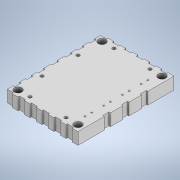
# Autodesk Inventor part: TOP_PANEL
Saved by Autodesk Inventor 2020.4 (Build 244396010, 396A)
## iProperties
Created: 2021-10-02
Part Number: TOP_PANEL
Material: Generic
Document SubType Name: Modeling
Designer: YUSTE
Density: 1 g/cm^3
Appearance: Default
Author: YUSTE
Autodesk Inventor part; units mm, degrees
ref_plane "YZ Plane" through (0, 0, 0) normal (1, 0, 0) x (0, 1, 0)
ref_plane "XZ Plane" through (0, 0, 0) normal (0, 1, 0) x (-1, 0, 0)
ref_plane "XY Plane" through (0, 0, 0) normal (0, 0, 1) x (1, 0, 0)
sketch "Sketch1" plane through (0, 0, 0) normal (0, 1, 0) x (-1, 0, 0)
  line L0 (0, 0) -> (152.4, 0)
  line L1 (152.4, 0) -> (152.4, 203.2)
  line L2 (152.4, 203.2) -> (0, 203.2)
  line L3 (0, 203.2) -> (0, 0)
  circle A0 centre (12.7, 190.5) radius 7.9375
  circle A1 centre (139.7, 190.5) radius 7.9375
  circle A2 centre (139.7, 12.7) radius 7.9375
  circle A3 centre (12.7, 12.7) radius 7.9375
  circle A4 centre (114.3, 190.5) radius 3.302
  circle A5 centre (38.1, 190.5) radius 3.302
  circle A6 centre (114.3, 12.7) radius 3.302
  circle A7 centre (38.1, 12.7) radius 3.302
  circle A8 centre (139.7, 139.7) radius 3.302
  circle A9 centre (139.7, 63.5) radius 3.302
  circle A10 centre (20.32, 168.148) radius 1.524
  circle A11 centre (20.32, 153.924) radius 1.524
  circle A12 centre (20.32, 128.524) radius 1.524
  circle A13 centre (20.32, 114.3) radius 1.524
  circle A14 centre (20.32, 88.9) radius 1.524
  circle A15 centre (20.32, 74.676) radius 1.524
  circle A16 centre (20.32, 49.276) radius 1.524
  circle A17 centre (20.32, 35.052) radius 1.524
  line L4 (152.4, 203.2) -> (139.7, 203.2)
  line L5 (139.7, 203.2) -> (139.7, 200.025)
  line L6 (139.7, 200.025) -> (152.4, 200.025)
  line L7 (152.4, 200.025) -> (152.4, 203.2)
  line L8 (127, 203.2) -> (114.3, 203.2)
  line L9 (114.3, 203.2) -> (114.3, 200.025)
  line L10 (114.3, 200.025) -> (127, 200.025)
  line L11 (127, 200.025) -> (127, 203.2)
  line L12 (101.6, 203.2) -> (88.9, 203.2)
  line L13 (88.9, 203.2) -> (88.9, 200.025)
  line L14 (88.9, 200.025) -> (101.6, 200.025)
  line L15 (101.6, 200.025) -> (101.6, 203.2)
  line L16 (76.2, 203.2) -> (63.5, 203.2)
  line L17 (63.5, 203.2) -> (63.5, 200.025)
  line L18 (63.5, 200.025) -> (76.2, 200.025)
  line L19 (76.2, 200.025) -> (76.2, 203.2)
  line L20 (50.8, 203.2) -> (38.1, 203.2)
  line L21 (38.1, 203.2) -> (38.1, 200.025)
  line L22 (38.1, 200.025) -> (50.8, 200.025)
  line L23 (50.8, 200.025) -> (50.8, 203.2)
  line L24 (25.4, 203.2) -> (12.7, 203.2)
  line L25 (12.7, 203.2) -> (12.7, 200.025)
  line L26 (12.7, 200.025) -> (25.4, 200.025)
  line L27 (25.4, 200.025) -> (25.4, 203.2)
  line L28 (152.4, 0) -> (139.7, 0)
  line L29 (139.7, 0) -> (139.7, 3.175)
  line L30 (139.7, 3.175) -> (152.4, 3.175)
  line L31 (152.4, 3.175) -> (152.4, 0)
  line L32 (127, 0) -> (114.3, 0)
  line L33 (114.3, 0) -> (114.3, 3.175)
  line L34 (114.3, 3.175) -> (127, 3.175)
  line L35 (127, 3.175) -> (127, 0)
  line L36 (101.6, 0) -> (88.9, 0)
  line L37 (88.9, 0) -> (88.9, 3.175)
  line L38 (88.9, 3.175) -> (101.6, 3.175)
  line L39 (101.6, 3.175) -> (101.6, 0)
  line L40 (76.2, 0) -> (63.5, 0)
  line L41 (63.5, 0) -> (63.5, 3.175)
  line L42 (63.5, 3.175) -> (76.2, 3.175)
  line L43 (76.2, 3.175) -> (76.2, 0)
  line L44 (50.8, 0) -> (38.1, 0)
  line L45 (38.1, 0) -> (38.1, 3.175)
  line L46 (38.1, 3.175) -> (50.8, 3.175)
  line L47 (50.8, 3.175) -> (50.8, 0)
  line L48 (25.4, 0) -> (12.7, 0)
  line L49 (12.7, 0) -> (12.7, 3.175)
  line L50 (12.7, 3.175) -> (25.4, 3.175)
  line L51 (25.4, 3.175) -> (25.4, 0)
  line L52 (152.4, 187.325) -> (149.225, 187.325)
  line L53 (149.225, 187.325) -> (149.225, 174.625)
  line L54 (149.225, 174.625) -> (152.4, 174.625)
  line L55 (152.4, 174.625) -> (152.4, 187.325)
  line L56 (152.4, 161.925) -> (149.225, 161.925)
  line L57 (149.225, 161.925) -> (149.225, 149.225)
  line L58 (149.225, 149.225) -> (152.4, 149.225)
  line L59 (152.4, 149.225) -> (152.4, 161.925)
  line L60 (152.4, 136.525) -> (149.225, 136.525)
  line L61 (149.225, 136.525) -> (149.225, 123.825)
  line L62 (149.225, 123.825) -> (152.4, 123.825)
  line L63 (152.4, 123.825) -> (152.4, 136.525)
  line L64 (152.4, 107.95) -> (149.225, 107.95)
  line L65 (149.225, 107.95) -> (149.225, 95.25)
  line L66 (149.225, 95.25) -> (152.4, 95.25)
  line L67 (152.4, 95.25) -> (152.4, 107.95)
  line L68 (152.4, 79.375) -> (149.225, 79.375)
  line L69 (149.225, 79.375) -> (149.225, 66.675)
  line L70 (149.225, 66.675) -> (152.4, 66.675)
  line L71 (152.4, 66.675) -> (152.4, 79.375)
  line L72 (152.4, 53.975) -> (149.225, 53.975)
  line L73 (149.225, 53.975) -> (149.225, 41.275)
  line L74 (149.225, 41.275) -> (152.4, 41.275)
  line L75 (152.4, 41.275) -> (152.4, 53.975)
  line L76 (152.4, 28.575) -> (149.225, 28.575)
  line L77 (149.225, 28.575) -> (149.225, 15.875)
  line L78 (149.225, 15.875) -> (152.4, 15.875)
  line L79 (152.4, 15.875) -> (152.4, 28.575)
  line L80 (0, 147.574) -> (0, 134.874)
  line L81 (0, 134.874) -> (3.175, 134.874)
  line L82 (3.175, 134.874) -> (3.175, 147.574)
  line L83 (3.175, 147.574) -> (0, 147.574)
  line L84 (0, 107.95) -> (0, 95.25)
  line L85 (0, 95.25) -> (3.175, 95.25)
  line L86 (3.175, 95.25) -> (3.175, 107.95)
  line L87 (3.175, 107.95) -> (0, 107.95)
  line L88 (0, 55.626) -> (0, 68.326)
  line L89 (0, 68.326) -> (3.175, 68.326)
  line L90 (3.175, 68.326) -> (3.175, 55.626)
  line L91 (3.175, 55.626) -> (0, 55.626)
  dimension "d0" = 152.4
  dimension "d1" = 203.2
  dimension "d40" = 15.875
  dimension "d41" = 15.875
  dimension "d42" = 15.875
  dimension "d43" = 15.875
  dimension "d44" = 12.7
  dimension "d45" = 12.7
  dimension "d46" = 12.7
  dimension "d47" = 12.7
  dimension "d48" = 12.7
  dimension "d49" = 12.7
  dimension "d50" = 12.7
  dimension "d51" = 12.7
  dimension "d52" = 177.8
  dimension "d53" = 127
  dimension "d54" = 6.604
  dimension "d55" = 6.604
  dimension "d56" = 25.4
  dimension "d57" = 25.4
  dimension "d58" = 12.7
  dimension "d59" = 12.7
  dimension "d60" = 6.604
  dimension "d61" = 6.604
  dimension "d62" = 12.7
  dimension "d63" = 12.7
  dimension "d64" = 25.4
  dimension "d65" = 25.4
  dimension "d66" = 6.604
  dimension "d67" = 6.604
  dimension "d68" = 50.8
  dimension "d69" = 50.8
  dimension "d70" = 12.7
  dimension "d71" = 12.7
  dimension "d72" = 3.048
  dimension "d73" = 3.048
  dimension "d74" = 3.048
  dimension "d75" = 3.048
  dimension "d76" = 3.048
  dimension "d77" = 3.048
  dimension "d78" = 20.32
  dimension "d79" = 20.32
  dimension "d80" = 20.32
  dimension "d81" = 20.32
  dimension "d82" = 20.32
  dimension "d83" = 20.32
  dimension "d84" = 22.352
  dimension "d85" = 14.224
  dimension "d86" = 25.4
  dimension "d87" = 14.224
  dimension "d88" = 25.4
  dimension "d89" = 14.224
  dimension "d90" = 3.048
  dimension "d91" = 3.048
  dimension "d92" = 25.4
  dimension "d93" = 14.224
  dimension "d97" = 12.7
  dimension "d98" = 3.175
  dimension "d99" = 12.7
  dimension "d100" = 3.175
  dimension "d101" = 12.7
  dimension "d102" = 3.175
  dimension "d103" = 12.7
  dimension "d104" = 3.175
  constraints: 180 end point, 45 parallel, 28 perpendicular, 18 centre point, 12 point on line, 1 horizontal, 1 vertical, 28 other
  measures "d0" distance of L3.start L1.end
  measures "d1" distance of L1.end L1.start
  measures "d40" diameter of A0
  measures "d41" diameter of A1
  measures "d42" diameter of A2
  measures "d43" diameter of A3
  measures "d45" distance from line of L3 A0.centre
  measures "d47" distance from line of L3 A3.centre
  measures "d49" distance from line of L1 A1.centre
  measures "d50" distance from line of L1 A2.centre
  measures "d52" distance of A2.centre A1.centre
  measures "d53" distance of A0.centre A1.centre
  measures "d54" diameter of A4
  measures "d55" diameter of A5
  measures "d56" distance of A0.centre A5.centre
  measures "d57" distance of A1.centre A4.centre
  measures "d60" diameter of A6
  measures "d61" diameter of A7
  measures "d64" distance of A2.centre A6.centre
  measures "d65" distance of A3.centre A7.centre
  measures "d66" diameter of A8
  measures "d67" diameter of A9
  measures "d68" distance of A1.centre A8.centre
  measures "d69" distance of A2.centre A9.centre
  measures "d70" distance from line of L1 A8.centre
  measures "d71" distance from line of L1 A9.centre
  measures "d72" diameter of A10
  measures "d73" diameter of A11
  measures "d74" diameter of A12
  measures "d75" diameter of A13
  measures "d76" diameter of A14
  measures "d77" diameter of A15
  measures "d78" distance from line of L3 A10.centre
  measures "d79" distance from line of L3 A11.centre
  measures "d80" distance from line of L3 A12.centre
  measures "d81" distance from line of L3 A13.centre
  measures "d82" distance from line of L3 A14.centre
  measures "d83" distance from line of L3 A15.centre
  measures "d84" vertical distance of A10.centre A0.centre
  measures "d85" distance of A10.centre A11.centre
  measures "d86" distance of A11.centre A12.centre
  measures "d87" distance of A12.centre A13.centre
  measures "d88" distance of A14.centre A13.centre
  measures "d89" distance of A14.centre A15.centre
  measures "d90" diameter of A16
  measures "d91" diameter of A17
  measures "d92" distance of A16.centre A15.centre
  measures "d93" distance of A16.centre A17.centre
  measures "d97" distance of L1.end L4.end
  measures "d98" distance of L5.end L4.end
  measures "d99" distance of L8.start L8.end
  measures "d100" distance of L9.end L8.end
  measures "d101" distance of L12.start L12.end
  measures "d102" distance of L13.end L12.end
  measures "d103" distance of L16.start L16.end
  measures "d104" distance of L17.end L16.end
extrude "Extrusion4" add sketch "Sketch1" along normal blind 25.4 contours L3 L91 L90 L89 L85 L86 L87 L81 L82 L83 L2 L25 L26 L27 L21 L22 L23 L17 L18 L19 L13 L14 L15 L9 L10 L11 L5 L6 L1 L52 L53 L54 L56 L57 L58 L60 L61 L62 L64 L65 L66 L68 L69 L70 L72 L73 L74 L76 L77 L78 L30 L29 L0 L35 L34 L33 L39 L38 L37 L43 L42 L41 L47 L46 L45 L51 L50 L49
body "Solid4"
